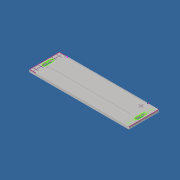
# Autodesk Inventor part: Fixture Base
Saved by Autodesk Inventor 2016 (Build 200138000, 138)
## iProperties
Created: 2016-04-07
Part Number: Fixture Base
Material: Generic
Document SubType Name: Modeling
Designer: Sam Clay
Density: 1 g/cm^3
Appearance: Default
Author: Sam Clay
Autodesk Inventor part; units mm, degrees
ref_plane "YZ Plane" through (0, 0, 0) normal (1, 0, 0) x (0, 1, 0)
ref_plane "XZ Plane" through (0, 0, 0) normal (0, 1, 0) x (-1, 0, 0)
ref_plane "XY Plane" through (0, 0, 0) normal (0, 0, 1) x (1, 0, 0)
sketch "Sketch1" plane through (0, 0, 0) normal (0, 1, 0) x (-1, 0, 0)
  line L0 (0, 0) -> (635, 0)
  line L1 (635, 0) -> (635, 228.6)
  line L2 (635, 228.6) -> (0, 228.6)
  line L3 (0, 228.6) -> (0, 0)
  line L4 (0, 228.6) -> (-76.2, 228.6)
  line L5 (-76.2, 228.6) -> (-76.2, 0)
  line L6 (-76.2, 0) -> (0, 0)
  line L7 (0, 0) -> (0, 228.6)
  line L8 (635, 228.6) -> (685.8, 228.6)
  line L9 (685.8, 228.6) -> (685.8, 0)
  line L10 (685.8, 0) -> (635, 0)
  line L11 (635, 0) -> (635, 228.6)
  dimension "d0" = 635
  dimension "d1" = 228.6
  dimension "d87" = 76.2
  dimension "d88" = 50.8
  constraints: 24 end point, 6 parallel, 3 horizontal, 3 perpendicular, 1 point on line
  measures "d0" distance of L2.end L1.end
  measures "d1" distance of L1.end L0.end
  measures "d87" distance of L6.end L5.end
  measures "d88" distance of L9.end L10.end
extrude "Extrusion1" add sketch "Sketch1" along normal blind 19.05 contours L3 L2 L1 L0
sketch "Sketch2" plane through (0, 19.05, 0) normal (0, 1, 0) x (1, 0, 0)
  line L0 (0, 0) -> (-635, 0) projected
  line L1 (-635, 0) -> (-635, -228.6) projected
  line L2 (0, 0) -> (-635, 0)
  line L3 (-635, 0) -> (-635, -20.066)
  line L4 (-635, -20.066) -> (0, -20.066)
  line L5 (0, -20.066) -> (0, 0)
  line L6 (0, 0) -> (-12.7, 0)
  line L7 (-12.7, 0) -> (-12.7, -121.666)
  line L8 (-12.7, -121.666) -> (0, -121.666)
  line L9 (0, -121.666) -> (0, 0)
  line L10 (-12.7, -154.178) -> (-635, -154.178)
  line L11 (-635, -154.178) -> (-635, -134.366)
  line L12 (-635, -134.366) -> (-12.7, -134.366)
  line L13 (-12.7, -134.366) -> (-12.7, -154.178)
  line L14 (0, -45.466) -> (-635, -45.466)
  line L15 (-635, -45.466) -> (-635, -32.766)
  line L16 (-635, -32.766) -> (0, -32.766)
  line L17 (0, -32.766) -> (0, -45.466)
  line L18 (-12.7, -42.506) -> (-9.74, -45.466)
  line L19 (-12.7, -42.506) -> (-16.886, -42.506) construction
  circle A0 centre (-17.3295, -50.0955) radius 8.89
  line L20 (-635, -0.254) -> (0, -0.254)
  line L21 (0, -228.6) -> (0, 0) projected
  line L22 (-12.7, -121.666) -> (-635, -121.666)
  line L23 (-635, -157.353) -> (0, -157.353)
  line L24 (-12.7, -154.178) -> (0, -154.178)
  line L25 (-12.7, -134.366) -> (0, -134.366)
  point P0 (-12.7, -20.066)
  point P1 (-12.7, -45.466)
  point P2 (-12.7, -45.466)
  dimension "d5" = 12.7
  dimension "d75" = 19.812
  dimension "d76" = 12.7
  dimension "d77" = 12.7
  dimension "d78" = 12.7
  dimension "d79" = 76.2
  dimension "d83" = 135
  dimension "d84" = 17.78
  dimension "d101" = 0.254
  dimension "d102" = 19.812
  dimension "d109" = 3.175
  constraints: 46 end point, 18 point on line, 8 parallel, 8 perpendicular, 6 horizontal, 3 coincident, 2 point on circle, 1 centre point, 1 equal length
  measures "d5" distance of L8.end L7.end
  measures "d75" distance of L10.end L11.end
  measures "d76" distance from line of L8.end L12
  measures "d77" distance of L14.end L15.end
  measures "d78" distance between parallel lines of L4 L16
  measures "d79" distance from line of L14 L7.end
  measures "d83" angle of L19 L18
  measures "d84" diameter of A0
  measures "d101" distance between parallel lines of L0 L20
  measures "d102" distance between parallel lines of L4 L20
  measures "d109" distance between parallel lines of L23 L10
extrude "Extrusion12" cut sketch "Sketch2" against normal blind 0.0254 contours L21 L23 L1 L10 L24
extrude "Extrusion2" cut sketch "Sketch2" against normal blind 3.175 contours L18 L14 L7 | A0 L18 | L7 L14 A0 | A0 L7 L14 | L14 A0 L7 L22 L1 | L7 A0 L14
extrude "Extrusion10" cut sketch "Sketch2" against normal blind 7.62 contours L5 L20 L7 L0 | L5 L4 L7 L20 | L7 L4 L1 L20 | L21 L24 L13 L25 | L13 L10 L1 L12
extrude "Extrusion11" add sketch "Sketch1" along normal blind 17.78 contours L6 L5 L4 L3 | L1 L8 L9 L10
sketch "Sketch8" plane through (0, 17.78, 0) normal (0, 1, 0) x (1, 0, 0)
  line L0 (-635, 0) -> (-685.8, 0) projected
  line L1 (-685.8, 0) -> (-685.8, -228.6) projected
  line L2 (76.2, -228.6) -> (76.2, 0) projected
  line L3 (-685.8, -228.6) -> (-635, -228.6) projected
  line L4 (50.8, -83.6181) -> (50.8, -142.6126) construction
  line L5 (38.1, -83.6181) -> (38.1, -142.6126)
  line L6 (63.5, -142.6126) -> (63.5, -83.6181)
  arc A0 (63.5, -83.6181) -> (38.1, -83.6181) centre (50.8, -83.6181) ccw
  arc A1 (38.1, -142.6126) -> (63.5, -142.6126) centre (50.8, -142.6126) ccw
  line L7 (-660.4, -83.6181) -> (-660.4, -142.6126) construction
  line L8 (-673.1, -83.6181) -> (-673.1, -142.6126)
  line L9 (-647.7, -142.6126) -> (-647.7, -83.6181)
  arc A2 (-647.7, -83.6181) -> (-673.1, -83.6181) centre (-660.4, -83.6181) ccw
  arc A3 (-673.1, -142.6126) -> (-647.7, -142.6126) centre (-660.4, -142.6126) ccw
  point P0 (0, 0)
  point P1 (-660.4, -25.4)
  point P2 (-660.4, -63.5)
  point P3 (-660.4, -165.1)
  point P4 (-622.3, 0)
  point P5 (50.8, -203.2)
  point P6 (50.8, -165.1)
  point P7 (50.8, -25.4)
  point P8 (-660.4, -203.2)
  point P9 (50.8, -63.5)
  point P10 (50.8, -113.1154)
  point P11 (-660.4, -113.1154)
  dimension "d91" = 25.4
  dimension "d97" = 38.1
  dimension "d99" = 38.1
  dimension "d100" = 25.4
  dimension "d103" = 25.4
  dimension "d104" = 25.4
  dimension "d105" = 25.4
  dimension "d106" = 25.4
  dimension "d107" = 25.4
  dimension "d108" = 25.4
  dimension "d114" = 12.7
  dimension "d115" = 25.4
  constraints: 16 end point, 8 point on circle, 8 tangent, 4 centre point, 2 midpoint, 2 parallel, 2 vertical, 2 vertical alignment
  measures "d91" distance from line of point (-660.4, -25.4) L0
  measures "d97" distance of point (-660.4, -63.5) point (-660.4, -25.4)
  measures "d99" distance of point (-660.4, -165.1) point (-660.4, -203.2)
  measures "d100" distance from line of L3 point (-660.4, -203.2)
  measures "d103" distance from line of point (-660.4, -63.5) L1
  measures "d104" distance from line of L1 point (-660.4, -25.4)
  measures "d105" distance from line of L1 point (-660.4, -165.1)
  measures "d106" distance from line of L1 point (-660.4, -203.2)
  measures "d107" distance from line of L2 point (50.8, -25.4)
  measures "d108" distance from line of L2 point (50.8, -63.5)
  measures "d114" distance between parallel lines of L6 L4
  measures "d115" diameter of A3
sketch "Sketch9" plane through (0, 19.05, 0) normal (0, 1, 0) x (1, 0, 0)
  point P0 (0, 0)
  point P1 (-12.7, -45.466)
  point P2 (-12.7, -45.466)
  constraints: 1 coincident
extrude "Extrusion13" cut sketch "Sketch8" against normal through all
equation "\"d104\" = d103"
equation "\"d105\" = d103"
equation "\"d106\" = d103"
equation "\"d107\" = d103"
equation "\"d108\" = d103"
body "Solid1"
